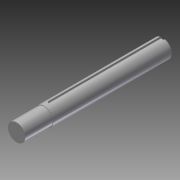
# Autodesk Inventor part: P80 Shaft (3.25 inch)
Saved by Autodesk Inventor 2013 (Build 170138000, 138)
## iProperties
Created: 2013-02-10
Part Number: P80 Shaft (3.25 inch)
Material: Steel
Document SubType Name: Modeling
Designer: Moses
Density: 7.85 g/cm^3
Mass: 94.2207 g
Surface Area: 46.5365 cm^2
Volume: 12.0026 cm^3
Author: Moses
Autodesk Inventor part; units mm, degrees
ref_plane "YZ Plane" through (0, 0, 0) normal (1, 0, 0) x (0, 1, 0)
ref_plane "XZ Plane" through (0, 0, 0) normal (0, 1, 0) x (-1, 0, 0)
ref_plane "XY Plane" through (0, 0, 0) normal (0, 0, 1) x (1, 0, 0)
sketch "Sketch1" plane through (0, 0, 0) normal (0, 0, 1) x (1, 0, 0)
  circle A0 centre (0, 0) radius 6.35
  circle A1 centre (0, 0) radius 2.3495
  dimension "d0" = 12.7
  dimension "d2" = 4.699
  constraints: 2 centre point, 2 coincident
  measures "d0" diameter of A0
  measures "d2" diameter of A1
extrude "Extrusion1" add sketch "Sketch1" along normal blind 82.55 contours A0 | A1
extrude "Extrusion2" cut sketch "Sketch1" along normal blind 12.7 contours A1
sketch "Sketch2" plane through (0, 0, 82.55) normal (0, 0, 1) x (1, 0, 0)
  circle A0 centre (0, 0) radius 6.35 projected
  circle A1 centre (0, 0) radius 6
  dimension "d7" = 12
  constraints: 1 centre point, 1 coincident
  measures "d7" diameter of A1
extrude "Extrusion3" add sketch "Sketch2" along normal blind 19.05 contours A1
sketch "Sketch3" plane through (0, 0, 0) normal (0, 0, -1) x (-1, 0, 0)
  circle A0 centre (0, 0) radius 6.35 projected
  line L0 (-1.5875, 6.1484) -> (-1.5875, 4.7625)
  line L1 (-1.5875, 4.7625) -> (1.5875, 4.7625)
  line L2 (1.5875, 4.7625) -> (1.5875, 6.1484)
  line L3 (0, 0) -> (0, 6.35) construction
  point P0 (0, 4.7625)
  dimension "d11" = 3.175
  dimension "d13" = 1.5875
  constraints: 8 end point, 3 point on circle, 1 midpoint, 1 parallel, 1 perpendicular, 1 point on line, 1 vertical
  measures "d11" distance of L0.end L1.end
  measures "d13" distance of L3.end point (0, 4.763)
extrude "Extrusion4" cut sketch "Sketch3" against normal blind 79.375 contours L2 L1 L0 A0 picked at (0.1781, 5.2842)
fillet "Fillet1" radius 1.5875 2 edges at (-1.5875, 5.4554, 79.375) (1.5875, 5.4554, 79.375)
chamfer "Chamfer1" distance 0.635 angle 45 2 edges at (5.0201, 3.8886, 0) (-3.8886, -5.0201, 0)
thread "Thread1" size "10-32 UNF" class "2B" standard "ANSI Unified Screw Threads" full length
body "Solid1"
